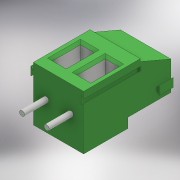
# Autodesk Inventor part: bornier_vert_5.08_variable
Saved by Autodesk Inventor 2018 (Build 220112000, 112)
## iProperties
Created: 2018-10-15
Part Number: bornier_vert_5.08_variable
Material: Générique
Document SubType Name: Modeling
Designer: Sébastien
Density: 1 g/cm^3
Appearance: Par défaut
Author: Sébastien
Autodesk Inventor part; units mm, degrees
ref_plane "YZ Plane" through (0, 0, 0) normal (1, 0, 0) x (0, 1, 0)
ref_plane "XZ Plane" through (0, 0, 0) normal (0, 1, 0) x (-1, 0, 0)
ref_plane "XY Plane" through (0, 0, 0) normal (0, 0, 1) x (1, 0, 0)
sketch "Esquisse1" plane through (0, 0, 0) normal (0, 1, 0) x (-1, 0, 0)
  circle A0 centre (0, 0) radius 0.525
  line L0 (2.65, -5.9) -> (-2.65, -5.9)
  line L1 (-2.65, -5.9) -> (-2.65, 5.3)
  line L2 (-2.65, 5.3) -> (2.65, 5.3)
  line L3 (2.65, 5.3) -> (2.65, -5.9)
  point P0 (0, 5.3)
  dimension "d0" = 1.05
  dimension "d1" = 11.2
  dimension "d2" = 5.3
  dimension "d4" = 2.65
  constraints: 8 end point, 2 coincident, 2 parallel, 1 centre point, 1 horizontal, 1 midpoint, 1 perpendicular, 1 vertical alignment
  measures "d0" diameter of A0
  measures "d1" distance of L0.end L1.end
  measures "d2" distance from line of A0.centre L2
  measures "d4" distance from line of L3 A0.centre
extrude "Extrusion1" add sketch "Esquisse1" along normal blind 18 contours A0 | L0 L1 L2 L3
sketch "Esquisse8" plane through (0, 0, 0) normal (0, 1, 0) x (-1, 0, 0)
  line L0 (-7.73, 3.1) -> (-7.23, 2.6)
  line L1 (-7.23, 2.6) -> (-7.23, 4.4)
  line L2 (-7.23, 4.4) -> (-7.73, 3.9)
  line L3 (-7.73, 3.9) -> (-7.73, 3.1)
  line L4 (2.65, 3.1) -> (3.15, 2.6)
  line L5 (3.15, 2.6) -> (3.15, 4.4)
  line L6 (3.15, 4.4) -> (2.65, 3.9)
  line L7 (2.65, 3.9) -> (2.65, 3.1)
  line L8 (-8.23, -0.95) -> (-8.23, -2.75)
  line L9 (-8.23, -2.75) -> (-7.73, -2.25)
  line L10 (-7.73, -2.25) -> (-7.73, -1.45)
  line L11 (-7.73, -1.45) -> (-8.23, -0.95)
  line L12 (2.15, -0.95) -> (2.15, -2.75)
  line L13 (2.15, -2.75) -> (2.65, -2.25)
  line L14 (2.65, -2.25) -> (2.65, -1.45)
  line L15 (2.65, -1.45) -> (2.15, -0.95)
  line L16 (0, 0) -> (0, -11.21) construction
  dimension "d45" = 45
  dimension "d46" = 0.8
  dimension "d47" = 1.8
  dimension "d48" = 4.4
  dimension "d49" = 45
  dimension "d50" = 0.8
  dimension "d51" = 1.8
  dimension "d53" = 7.73
  dimension "d56" = 2.65
  dimension "d105" = 1.8
  dimension "d106" = 45
  dimension "d107" = 0.8
  dimension "d108" = 135
  dimension "d109" = 1.8
  dimension "d110" = 45
  dimension "d111" = 0.8
  dimension "d112" = 135
  dimension "d119" = 2.75
  constraints: 36 end point, 5 vertical, 4 parallel, 2 horizontal alignment, 2 perpendicular, 2 vertical alignment
  measures "d45" angle of L1 L0
  measures "d46" distance of L2.end L0.start
  measures "d47" distance of L0.end L1.end
  measures "d48" vertical distance of L1.end L16.start
  measures "d49" angle of L5 L4
  measures "d50" distance of L6.end L4.start
  measures "d51" distance of L4.end L5.end
  measures "d53" distance from line of L16.start L3
  measures "d56" distance from line of L16.start L7
  measures "d105" distance of L8.start L8.end
  measures "d106" angle of L9 L8
  measures "d107" distance of L9.end L10.end
  measures "d108" angle of L11 L10
  measures "d109" distance of L12.start L12.end
  measures "d110" angle of L13 L12
  measures "d111" distance of L13.end L14.end
  measures "d112" angle of L15 L14
  measures "d119" vertical distance of L16.start L12.end
sketch "Esquisse9" plane through (0, 18, 0) normal (0, 1, 0) x (1, 0, 0)
  line L0 (-2.15, 2.75) -> (-2.65, 2.25) projected
  line L1 (-2.65, 2.25) -> (-2.65, 1.45) projected
  line L2 (-2.15, 0.95) -> (-2.15, 2.75) projected
  line L3 (-2.65, 1.45) -> (-2.15, 0.95) projected
  line L4 (8.23, 2.75) -> (7.73, 2.25) projected
  line L5 (8.23, 0.95) -> (8.23, 2.75) projected
  line L6 (7.73, 1.45) -> (8.23, 0.95) projected
  line L7 (7.73, 2.25) -> (7.73, 1.45) projected
sketch "Esquisse2" plane through (2.65, 0, 5.3) normal (1, 0, 0) x (0, 0, -1)
  line L0 (11.2, 0) -> (0, 0) projected
  line L1 (11.2, 0) -> (11.2, 18) construction
  line L2 (0, 18) -> (11.2, 18) construction
  line L3 (0, 0) -> (0, 18) construction
  line L4 (3.2, 18) -> (9.2, 18)
  line L5 (9.2, 18) -> (9.2, 9.1)
  line L6 (9.2, 9.1) -> (11.2, 9.1)
  line L7 (0, 11.7) -> (0.52, 11.7)
  line L8 (0.52, 11.7) -> (3.2, 18)
  line L9 (0, 11.7) -> (0, 18)
  line L10 (0, 18) -> (3.2, 18)
  line L11 (9.2, 18) -> (11.2, 18)
  line L12 (11.2, 18) -> (11.2, 9.1)
  point P0 (5.3, 0)
  dimension "d7" = 0.52
  dimension "d8" = 6
  dimension "d9" = 9.1
  dimension "d10" = 2
  dimension "d11" = 11.7
  constraints: 18 end point, 4 point on line, 3 collinear, 3 perpendicular, 1 vertical
  measures "d7" distance of L7.start L7.end
  measures "d8" distance of L4.start L4.end
  measures "d9" distance between parallel lines of L0 L6
  measures "d10" distance of L5.end L6.end
  measures "d11" distance from line of L0 L7.start
extrude "Extrusion2" cut sketch "Esquisse2" against normal through all
sketch "Esquisse3" plane through (0, 18, 0) normal (0, 1, 0) x (1, 0, 0)
  line L0 (-2.65, -2.1) -> (2.65, -2.1) projected
  line L1 (2.65, -2.1) -> (2.65, 3.9) projected
  line L2 (2.65, 3.9) -> (-2.65, 3.9) projected
  line L3 (-2.65, 3.9) -> (-2.65, -2.1) projected
  circle A0 centre (0, 0.25) radius 1.95
  point P0 (0, 0)
  point P1 (0, -2.1)
  dimension "d14" = 3.9
  dimension "d15" = 1.7
  constraints: 1 centre point, 1 midpoint, 1 vertical alignment
  measures "d14" diameter of A0
  measures "d15" distance edge to line of A0 L2
extrude "Extrusion3" cut sketch "Esquisse3" against normal blind 1 contours A0
sketch "Esquisse4" plane through (0, 17, -0.25) normal (0, 1, 0) x (1, 0, 0)
  circle A0 centre (0, 0) radius 1.95 projected
  line L0 (-1.9085, 0.4) -> (1.9085, 0.4)
  line L1 (-1.9085, -0.4) -> (1.9085, -0.4)
  point P0 (0, -0.25)
  dimension "d18" = 0.8
  constraints: 4 end point, 4 point on circle, 2 parallel, 1 horizontal
  measures "d18" distance between parallel lines of L0 L1
extrude "Extrusion4" cut sketch "Esquisse4" against normal blind 0.5 contours A0 L1 L0
sketch "Esquisse5" plane through (-2.65, 0, 5.3) normal (0, 0, 1) x (1, 0, 0)
  line L0 (5.3, 11.7) -> (0, 11.7) projected
  line L1 (0, 0) -> (0, 11.7) projected
  line L2 (5.3, 0) -> (0, 0) projected
  line L3 (5.3, 0) -> (5.3, 11.7) projected
  line L4 (1.225, 8.5) -> (4.075, 8.5)
  line L5 (4.075, 8.5) -> (4.075, 2.7)
  line L6 (4.075, 2.7) -> (1.225, 2.7)
  line L7 (1.225, 2.7) -> (1.225, 8.5)
  point P0 (2.65, 0)
  dimension "d21" = 1.225
  dimension "d22" = 2.85
  dimension "d23" = 5.8
  dimension "d24" = 2.7
  dimension "d25" = 1.225
  constraints: 8 end point, 2 parallel, 1 horizontal, 1 perpendicular
  measures "d21" distance between parallel lines of L3 L5
  measures "d22" distance of L5.end L6.end
  measures "d23" distance of L4.end L5.end
  measures "d24" distance between parallel lines of L2 L6
  measures "d25" distance between parallel lines of L1 L7
extrude "Extrusion5" cut sketch "Esquisse5" against normal blind 2.77 contours L4 L5 L6 L7
chamfer "Chanfrein1" distance 0.5 angle 45 4 edges at (-1.425, 5.6, 5.3) (0, 8.5, 5.3) (1.425, 5.6, 5.3) (0, 2.7, 5.3)
sketch "Esquisse6" plane through (-2.65, 0, 2.53) normal (0, 0, 1) x (1, 0, 0)
  line L0 (1.225, 8.5) -> (4.075, 8.5) projected
  line L1 (1.225, 2.7) -> (1.225, 8.5) projected
  line L2 (4.075, 2.7) -> (1.225, 2.7) projected
  line L3 (4.075, 8.5) -> (4.075, 2.7) projected
  line L4 (1.225, 4.4) -> (4.075, 4.4)
  point P0 (2.65, 0)
  dimension "d31" = 1.7
  constraints: 2 end point, 2 point on line, 1 perpendicular
  measures "d31" distance between parallel lines of L2 L4
extrude "Extrusion6" cut sketch "Esquisse6" against normal blind 3 contours L0 L3 L4 L1
sketch "Esquisse7" plane through (2.65, 0, -5.9) normal (0, 0, -1) x (-1, 0, 0)
  line L0 (5.3, 9.1) -> (0, 9.1) construction
  line L1 (0, 0) -> (0, 9.1) construction
  line L2 (5.3, 0) -> (0, 0) construction
  line L3 (5.3, 0) -> (5.3, 9.1) construction
  line L4 (1.15, 9.1) -> (1.15, 5.1)
  line L5 (1.15, 5.1) -> (4.15, 5.1)
  line L6 (4.15, 5.1) -> (4.15, 9.1)
  line L7 (4.15, 9.1) -> (1.15, 9.1)
  point P0 (2.65, 0)
  dimension "d34" = 3
  dimension "d35" = 4
  dimension "d36" = 1.15
  dimension "d37" = 1.15
  constraints: 8 end point, 2 perpendicular, 2 point on line, 1 horizontal, 1 vertical
  measures "d34" distance of L4.end L5.end
  measures "d35" distance of L5.end L6.end
  measures "d36" distance between parallel lines of L3 L6
  measures "d37" distance between parallel lines of L1 L4
extrude "Extrusion7" cut sketch "Esquisse7" against normal blind 1.5
extrude "Extrusion8" add sketch "Esquisse1" against normal blind 5 contours A0
sketch "SilkS" plane through (0, 18, 0) normal (0, 1, 0) x (1, 0, 0)
  line L0 (2.65, -5.3) -> (-10.27, -5.3)
  line L1 (-10.27, 5.9) -> (2.65, 5.9)
  line L2 (-10.27, 5.9) -> (-10.27, -5.3)
  line L3 (2.65, 5.9) -> (2.65, -5.3)
  point P0 (0, 0)
  dimension "d121" = 10.27
  constraints: 8 end point, 2 coincident, 2 vertical, 1 horizontal, 1 perpendicular
  measures "d121" distance from line of point (0, 0) L2
sketch "CrtYd" plane through (0, 18, 0) normal (0, 1, 0) x (1, 0, 0)
  line L0 (7.73, -3.1) -> (7.23, -2.6) projected
  line L1 (7.23, -2.6) -> (7.23, -4.4) projected
  line L2 (7.73, -3.9) -> (7.73, -3.1) projected
  line L3 (7.23, -4.4) -> (7.73, -3.9) projected
  line L4 (-2.65, -3.1) -> (-3.15, -2.6) projected
  line L5 (-3.15, -2.6) -> (-3.15, -4.4) projected
  line L6 (-2.65, -3.9) -> (-2.65, -3.1) projected
  line L7 (-3.15, -4.4) -> (-2.65, -3.9) projected
  line L8 (2.65, 2.35) -> (2.65, 1.55) projected
  line L9 (3.15, 2.85) -> (2.65, 2.35) projected
  line L10 (3.15, 1.05) -> (3.15, 2.85) projected
  line L11 (2.65, 1.55) -> (3.15, 1.05) projected
  line L12 (-2.15, 2.85) -> (-2.65, 2.35) projected
  line L13 (-2.15, 1.05) -> (-2.15, 2.85) projected
  line L14 (-2.65, 2.35) -> (-2.65, 1.55) projected
  line L15 (-2.65, 1.55) -> (-2.15, 1.05) projected
  circle A0 centre (0, 0.25) radius 1.95 construction
  line L16 (1.425, -4.8) -> (-1.425, -4.8) construction
  line L17 (-1.925, -5.3) -> (-1.425, -4.8) construction
  line L18 (-1.925, -5.3) -> (1.925, -5.3) construction
  line L19 (1.925, -5.3) -> (1.425, -4.8) construction
  line L20 (1.425, -4.8) -> (-1.425, -4.8) construction
  line L21 (1.425, -4.8) -> (1.425, -2.53) construction
  line L22 (1.425, -2.53) -> (-1.425, -2.53) construction
  line L23 (-1.425, -4.8) -> (-1.425, -2.53) construction
  circle A1 centre (0, 0.25) radius 1.95
  line L24 (1.425, -2.53) -> (1.425, -4.8)
  line L25 (1.425, -4.8) -> (1.925, -5.3)
  line L26 (1.925, -5.3) -> (-1.925, -5.3)
  line L27 (-1.925, -5.3) -> (-1.425, -4.8)
  line L28 (-1.425, -4.8) -> (-1.425, -2.53)
  line L29 (-1.425, -2.53) -> (1.425, -2.53)
  line L30 (1.425, -4.8) -> (-1.425, -4.8)
  circle A2 centre (5.08, 0.25) radius 1.95
  line L31 (3.655, -2.53) -> (6.505, -2.53)
  line L32 (3.655, -4.8) -> (3.655, -2.53)
  line L33 (6.505, -2.53) -> (6.505, -4.8)
  line L34 (6.505, -4.8) -> (3.655, -4.8)
  line L35 (7.005, -5.3) -> (3.155, -5.3)
  line L36 (6.505, -4.8) -> (7.005, -5.3)
  line L37 (3.155, -5.3) -> (3.655, -4.8)
  line L38 (-2.65, -3.9) -> (-2.65, -5.3)
  line L39 (-2.65, -5.3) -> (7.73, -5.3)
  line L40 (7.73, -5.3) -> (7.73, -3.9)
  line L41 (2.65, -3.1) -> (2.65, 1.55)
  line L42 (2.65, 2.35) -> (2.65, 5.9)
  line L43 (2.65, 5.9) -> (-2.65, 5.9)
  line L44 (-2.65, 5.9) -> (-2.65, 2.35)
  line L45 (-2.65, 1.55) -> (-2.65, -3.1)
  point P0 (0, 0)
  dimension "d98" = 5.08
  constraints: 42 end point, 6 perpendicular, 4 collinear, 3 vertical, 2 centre point, 2 coincident, 1 concentric, 1 horizontal, 22 other
  measures "d98" distance of A1.centre A2.centre
pattern_linear "Réseau rectangulaire1" count 2 spacing 5.08 along (1, 0, 0)
extrude "Extrusion9" cut sketch "Esquisse8" along normal up to surface (11.7 mm away) contours L3 L2 L1 L0
extrude "Extrusion10" add sketch "Esquisse8" along normal up to surface (11.7 mm away) contours L7 L6 L5 L4
extrude "Extrusion11" add sketch "Esquisse9" against normal blind 2.9 contours L5 L6 L7 L4
extrude "Extrusion12" cut sketch "Esquisse9" against normal blind 2.9 contours L2 L3 L1 L0
equation "\"d21\" = d25"
equation "\"d36\" = d37"
